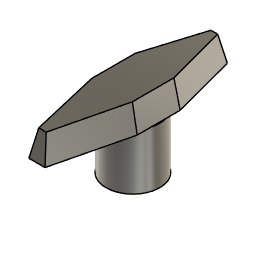
deadbold_knob v4 (Autodesk Fusion 360 design; units mm, degrees)
Autodesk Fusion 360 part; units mm, degrees
sketch "Sketch1" plane through (0, 0, 0) normal (0, 0, 1) x (1, 0, 0)
  circle A0 centre (0, 0) radius 6.25
  dimension "d1" = 12.5
  constraint coincident A0.centre origin
  measures "d1" diameter of A0
extrude "Extrude1" add sketch "Sketch1" along normal blind 13
sketch "Sketch2" plane through (0, 0, 13) normal (0, 0, 1) x (-1, 0, 0)
  circle A0 centre (0, 0) radius 6.25
  line L0 (6, -5.4238) -> (1.515, -20)
  line L1 (1.515, -20) -> (-2, -20)
  line L2 (-2, -20) -> (-6, -5)
  line L3 (-6, -5) -> (-6, 5)
  line L4 (-6, 5) -> (-1.8178, 22.2905)
  line L5 (-1.8178, 22.2905) -> (1.9317, 22.2905)
  line L6 (1.9317, 22.2905) -> (6, 5)
  line L7 (6, 5) -> (6, -5.4238)
  constraint horizontal L1
  constraint perpendicular L1 L3
  constraint perpendicular L3 L5
  constraint vertical L7
extrude "Extrude2" add sketch "Sketch2" along normal blind 6 draft -12 contours A0 L3 L7 | A0 L3 L4 L5 L6 L7 | A0 L0 L1 L2 L3 L7
